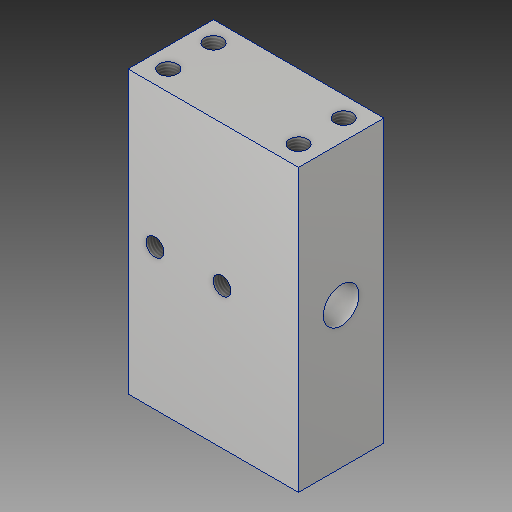
# Autodesk Inventor part: MotorMountRight
Saved by Autodesk Inventor 2019.3 (Build 233278000, 278)
## iProperties
Created: 2019-01-26
Part Number: MotorMountRight
Material: Aluminum 6061
Document SubType Name: Modeling
Designer: mark
Density: 2.7 g/cm^3
Appearance: Aluminum - Flat
Author: mark
Autodesk Inventor part; units mm, degrees
ref_plane "YZ Plane" through (0, 0, 0) normal (1, 0, 0) x (0, 1, 0)
ref_plane "XZ Plane" through (0, 0, 0) normal (0, 1, 0) x (-1, 0, 0)
ref_plane "XY Plane" through (0, 0, 0) normal (0, 0, 1) x (1, 0, 0)
sketch "Sketch1" plane through (0, 0, 0) normal (0, 0, 1) x (1, 0, 0)
  line L0 (0, 0) -> (76.2, 0)
  line L1 (76.2, 0) -> (76.2, 125.8)
  line L2 (76.2, 125.8) -> (0, 125.8)
  line L3 (0, 125.8) -> (0, 0)
  circle A0 centre (12, 62.9) radius 4
  circle A1 centre (42, 62.9) radius 4
  dimension "d0" = 76.2
  dimension "d1" = 125.8
  dimension "d2" = 8
  dimension "d3" = 8
  dimension "d4" = 12
  dimension "d5" = 42
  dimension "d6" = 62.9
  dimension "d7" = 62.9
  constraints: 8 end point, 2 centre point, 2 perpendicular, 1 horizontal
  measures "d0" distance of L2.end L1.end
  measures "d1" distance between parallel lines of L0 L2
  measures "d2" diameter of A0
  measures "d3" diameter of A1
  measures "d4" distance from line of L3 A0.centre
  measures "d5" distance from line of L3 A1.centre
  measures "d6" distance from line of L0 A1.centre
  measures "d7" distance from line of L0 A0.centre
extrude "Extrusion1" add sketch "Sketch1" along normal blind 38.2 contours L3 L2 L1 L0 | A0 | A1
sketch "Sketch2" plane through (0, 0, 38.2) normal (0, 0, 1) x (1, 0, 0)
  line L0 (0, 0) -> (76.2, 0)
  line L1 (76.2, 0) -> (76.2, 125.8)
  line L2 (76.2, 125.8) -> (0, 125.8)
  line L3 (0, 125.8) -> (0, 0)
  circle A0 centre (12, 62.9) radius 4
  circle A1 centre (42, 62.9) radius 4
  dimension "d17" = 76.2
  dimension "d16" = 125.8
  dimension "d13" = 8
  dimension "d10" = 8
  dimension "d15" = 12
  dimension "d12" = 42
  dimension "d11" = 62.9
  dimension "d14" = 62.9
  constraints: 8 end point, 2 centre point, 2 perpendicular, 1 horizontal
  measures "d17" distance of L2.end L1.end
  measures "d16" distance between parallel lines of L0 L2
  measures "d13" diameter of A0
  measures "d10" diameter of A1
  measures "d15" distance from line of L3 A0.centre
  measures "d12" distance from line of L3 A1.centre
  measures "d11" distance from line of L0 A1.centre
  measures "d14" distance from line of L0 A0.centre
extrude "Extrusion2" cut sketch "Sketch2" against normal blind 19.1 contours A0 | A1
sketch "Sketch3" plane through (0, 0, 0) normal (-1, 0, 0) x (0, 0, 1)
  circle A0 centre (19.1, 62.9) radius 8
  line L0 (38.2, 125.8) -> (38.2, 0) projected
  line L1 (0, 0) -> (38.2, 0) projected
  dimension "d21" = 16
  dimension "d22" = 19.1
  dimension "d23" = 62.9
  constraints: 1 centre point
  measures "d21" diameter of A0
  measures "d22" distance from line of L0 A0.centre
  measures "d23" distance from line of L1 A0.centre
extrude "Extrusion3" cut sketch "Sketch3" against normal up to next
thread "Thread1" size "M8x1.25" class "6H" standard "ANSI Metric M Profile" full length
thread "Thread2" size "M8x1.25" class "6H" standard "ANSI Metric M Profile" full length
sketch "Sketch4" plane through (0, 0, 0) normal (0, -1, 0) x (1, 0, 0)
  circle A0 centre (9, 29.2) radius 4
  circle A1 centre (9, 9) radius 4
  circle A2 centre (67.2, 29.2) radius 4
  circle A3 centre (67.2, 9) radius 4
  line L0 (0, 38.2) -> (76.2, 38.2) projected
  line L1 (0, 0) -> (0, 38.2) projected
  dimension "d33" = 8
  dimension "d34" = 8
  dimension "d35" = 8
  dimension "d36" = 8
  dimension "d41" = 20.2
  dimension "d42" = 58.2
  dimension "d45" = 20.2
  dimension "d46" = 58.2
  dimension "d48" = 9
  dimension "d49" = 9
  dimension "d51" = 9
  dimension "d52" = 9
  constraints: 4 centre point
  measures "d33" diameter of A0
  measures "d34" diameter of A1
  measures "d35" diameter of A2
  measures "d36" diameter of A3
  measures "d41" distance of A2.centre A3.centre
  measures "d42" distance of A1.centre A3.centre
  measures "d45" distance of A0.centre A1.centre
  measures "d46" distance of A0.centre A2.centre
  measures "d48" distance from line of A0.centre L0
  measures "d49" distance from line of L0 A2.centre
  measures "d51" distance from line of L1 A0.centre
  measures "d52" distance from line of L1 A1.centre
extrude "Extrusion4" cut sketch "Sketch4" against normal blind 30
sketch "Sketch5" plane through (0, 125.8, 38.2) normal (0, 1, 0) x (1, 0, 0)
  circle A0 centre (67.2, 29.2) radius 4
  circle A1 centre (67.2, 9) radius 4
  circle A2 centre (9, 29.2) radius 4
  circle A3 centre (9, 9) radius 4
  line L0 (0, 38.2) -> (76.2, 38.2)
  line L1 (0, 0) -> (0, 38.2)
  dimension "d56" = 8
  dimension "d55" = 8
  dimension "d64" = 8
  dimension "d63" = 8
  dimension "d65" = 20.2
  dimension "d59" = 58.2
  dimension "d58" = 20.2
  dimension "d62" = 58.2
  dimension "d61" = 9
  dimension "d66" = 9
  dimension "d60" = 9
  dimension "d57" = 9
  constraints: 4 centre point, 4 end point
  measures "d56" diameter of A2
  measures "d55" diameter of A3
  measures "d64" diameter of A0
  measures "d63" diameter of A1
  measures "d65" distance of A0.centre A1.centre
  measures "d59" distance of A3.centre A1.centre
  measures "d58" distance of A2.centre A3.centre
  measures "d62" distance of A2.centre A0.centre
  measures "d61" distance from line of A2.centre L0
  measures "d66" distance from line of L0 A0.centre
  measures "d60" distance from line of L1 A2.centre
  measures "d57" distance from line of L1 A3.centre
extrude "Extrusion5" cut sketch "Sketch5" against normal blind 30
thread "Thread3" size "M8x1.25" class "6H" standard "ANSI Metric M Profile" full length
thread "Thread4" size "M8x1.25" class "6H" standard "ANSI Metric M Profile" full length
thread "Thread5" size "M8x1.25" class "6H" standard "ANSI Metric M Profile" full length
thread "Thread6" size "M8x1.25" class "6H" standard "ANSI Metric M Profile" full length
thread "Thread7" size "M8x1.25" class "6H" standard "ANSI Metric M Profile" full length
thread "Thread8" size "M8x1.25" class "6H" standard "ANSI Metric M Profile" full length
thread "Thread9" size "M8x1.25" class "6H" standard "ANSI Metric M Profile" full length
thread "Thread10" size "M8x1.25" class "6H" standard "ANSI Metric M Profile" full length
body "Solid1"
